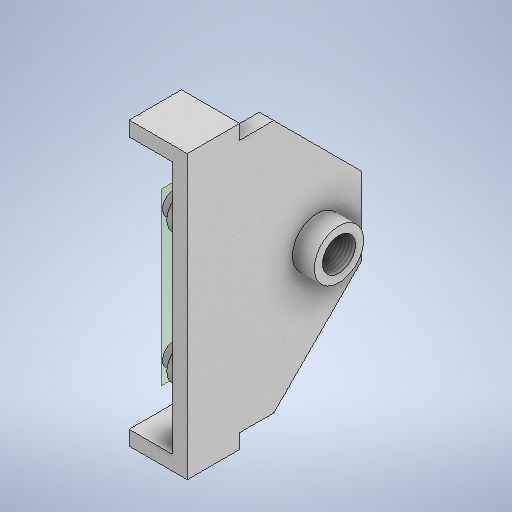
# Autodesk Inventor part: Führungsplatte_links
Saved by Autodesk Inventor 2025.2 (Build 292293000, 293)
## iProperties
Created: 2025-02-03
Part Number: Führungsplatte_links
Material: Generisch
Document SubType Name: Modeling
Designer: unter
Density: 1 g/cm^3
Appearance: 1-Zoll-Quadrate - Mosaik-Grau
Author: unter
Autodesk Inventor part; units mm, degrees
ref_plane "YZ Plane" through (0, 0, 0) normal (1, 0, 0) x (0, 1, 0)
ref_plane "XZ Plane" through (0, 0, 0) normal (0, 1, 0) x (-1, 0, 0)
ref_plane "XY Plane" through (0, 0, 0) normal (0, 0, 1) x (1, 0, 0)
derived "Skelett_Laufkatze.ipt"
sketch "Fuehrungsplatte_seite_ohne" plane through (116, 0, 0) normal (1, 0, 0) x (0, 1, 0)
  line L0 (174, 98.4) -> (-174, 98.4)
  line L1 (-174, 98.4) -> (-194, 98.4)
  line L2 (-194, 98.4) -> (-194, 26.4)
  line L3 (-194, 26.4) -> (-174, 26.4)
  line L4 (-174, 26.4) -> (-174, -20.4)
  line L5 (-174, -20.4) -> (-54, -140.4)
  line L6 (-54, -140.4) -> (54, -140.4)
  line L7 (54, -140.4) -> (174, -20.4)
  line L8 (174, 26.4) -> (174, -20.4)
  line L9 (194, 26.4) -> (174, 26.4)
  line L10 (194, 98.4) -> (194, 26.4)
  line L11 (174, 98.4) -> (194, 98.4)
  circle A0 centre (-90, 62.4) radius 54 construction
  circle A1 centre (90, 62.4) radius 54 construction
  circle A2 centre (-90, 62.4) radius 25
  circle A3 centre (-90, 62.4) radius 15
  circle A4 centre (90, 62.4) radius 25
  circle A5 centre (90, 62.4) radius 15
  circle A6 centre (0, -80) radius 33.75
  circle A7 centre (0, -80) radius 22.5
  point P0 (0, 0)
sketch "Fuehrungsplatte_Laufradaufhängung_ohne" plane through (116, -90, 62.4) normal (0, 0, -1) x (-1, 0, 0)
  line L0 (0, 25) -> (0, -25)
  line L1 (0, 15) -> (0, -15)
  line L2 (0, 205) -> (0, 155)
  line L3 (0, 195) -> (0, 165)
  line L4 (0, 205) -> (19, 205)
  line L5 (19, 205) -> (19, 155)
  line L6 (19, 155) -> (0, 155)
  line L7 (19, 195) -> (35, 195)
  line L8 (35, 195) -> (35, 165)
  line L9 (35, 165) -> (19, 165)
  line L10 (0, 25) -> (19, 25)
  line L11 (19, 25) -> (19, -25)
  line L12 (19, -25) -> (0, -25)
  line L13 (19, 15) -> (35, 15)
  line L14 (35, 15) -> (35, -15)
  line L15 (35, -15) -> (19, -15)
  line L16 (247, 284) -> (267, 284) construction
  line L17 (247, 264) -> (247, 284) construction
  line L18 (267, -104) -> (247, -104) construction
  line L19 (247, -84) -> (247, -104) construction
  line L20 (0, 284) -> (-20, 284)
  line L21 (-20, 284) -> (-20, -104)
  line L22 (-20, -104) -> (0, -104)
  line L23 (0, -104) -> (0, 284)
  line L24 (0, -104) -> (60, -104)
  line L25 (60, -104) -> (60, -84)
  line L26 (60, -84) -> (0, -84)
  line L27 (0, -84) -> (0, -104)
  line L28 (0, 284) -> (60, 284)
  line L29 (60, 284) -> (60, 264)
  line L30 (60, 264) -> (0, 264)
  line L31 (0, 264) -> (0, 284)
  point P0 (116, 90)
  point P1 (35, 0)
  point P2 (35, 180)
sketch "Fuehrungsplatte_Schraubbolzen_ohne" plane through (116, 0, -80) normal (0, 0, -1) x (-1, 0, 0)
  line L0 (0, 33.75) -> (0, -33.75)
  line L1 (0, 22.5) -> (0, -22.5)
  line L2 (0, 33.75) -> (-50, 33.75)
  line L3 (-50, 33.75) -> (-50, -33.75)
  line L4 (-50, -33.75) -> (0, -33.75)
  line L5 (0, 22.5) -> (-50, 22.5)
  line L6 (0, -22.5) -> (-50, -22.5)
  point P0 (116, 0)
extrude "Grundplatte" add sketch "Fuehrungsplatte_seite_ohne" along normal up to surface (20 mm away) contours L11 L10 L9 L8 L7 L6 L5 L4 L3 L2 L1 L0
extrude "Schutzwände" add sketch "Fuehrungsplatte_Laufradaufhängung_ohne" against normal up to surface (72 mm away) from surface at 36 contours L26 L25 L24 L23 | L23 L28 L29 L30
extrude "Laufradaufhängung_1" add sketch "Fuehrungsplatte_seite_ohne" against normal up to surface (39 mm away) from surface at 20 contours A4 | A5
extrude "Laufradaufhängung_2" add sketch "Fuehrungsplatte_seite_ohne" against normal up to surface (35 mm away) contours A5
extrude "Laufradaufhängung_3" add sketch "Fuehrungsplatte_seite_ohne" against normal up to surface (39 mm away) from surface at 20 contours A2 | A3
extrude "Laufradaufhängung_4" add sketch "Fuehrungsplatte_seite_ohne" against normal up to surface (35 mm away) contours A3
extrude "Schraubbolzenöffnung" add sketch "Fuehrungsplatte_seite_ohne" along normal up to surface (50 mm away) from surface at 0 contours A6
thread "Gewinde1" size "M45x4.5" class "6H" standard "ANSI Metric M Profile" full length
ref_plane "Arbeitsebene2" through (81, 90, 62.4) normal (-1, 0, 0) x (0, 0, 1)
sketch "Skizze5" plane through (81, 90, 62.4) normal (-1, 0, 0) x (0, 0, 1)
  circle A0 centre (0, 0) radius 15 projected
  circle A1 centre (0, -180) radius 15 projected
  point P0 (-62.4, -90)
  constraints: 2 coincident
hole "Bohrung1" at (81, 90, 62.4) at (81, -90, 62.4) direction (1, 0, 0) diameter 10.106 depth 32.3 tip angle 118 thread size "M12x1.75" class "6H" standard "ISO Metric profile"
